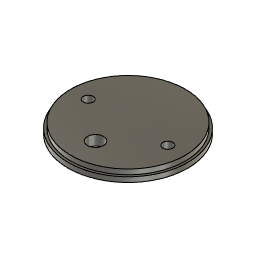
BulkPlate_Payload_AftMost_Subscalev1 (Autodesk Fusion 360 design; units mm, degrees)
Autodesk Fusion 360 part; units mm, degrees
sketch "Sketch1" plane through (0, 0, 0) normal (0, 0, 1) x (1, 0, 0)
  circle A0 centre (0, 0) radius 38.0746
  dimension "d1" = 76.1492
  constraint coincident A0.centre origin
  measures "d1" diameter of A0
extrude "Extrude1" add sketch "Sketch1" along normal blind 3.175
sketch "Sketch2" plane through (0, 0, 3.175) normal (0, 0, 1) x (-1, 0, 0)
  circle A0 centre (0, 0) radius 38.0746
  circle A1 centre (0, 0) radius 36.5125
  dimension "d4" = 73.025
  constraint coincident A0.centre A1.centre
  measures "d4" diameter of A1
extrude "Extrude2" add sketch "Sketch2" along normal blind 3.175 contours A1
sketch "Sketch3" plane through (0, 0, 6.35) normal (0, 0, 1) x (-1, 0, 0)
  circle A0 centre (0, 0) radius 36.5125
  circle A1 centre (25.4, 0) radius 3.175
  circle A2 centre (-25.4, 0) radius 3.175
  circle A3 centre (0, 20.6756) radius 5.08
  circle A4 centre (0, 0) radius 38.0746
  dimension "d7" = 6.35
  dimension "d8" = 6.35
  dimension "d9" = 50.8
  dimension "d10" = 25.4
  dimension "d11" = 10.16
  dimension "d12" = 20.6756
  measures "d7" diameter of A1
  measures "d8" diameter of A2
  measures "d9" distance of A1.centre A2.centre
  measures "d10" distance of A0.centre A2.centre
  measures "d11" diameter of A3
  measures "d12" distance of A3.centre A0.centre
extrude "Extrude3" cut sketch "Sketch3" against normal blind 22.86 contours A1 | A2 | A3
